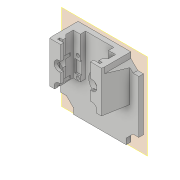
# Autodesk Inventor part: 50_Cube_Insert_Thorlabs
Saved by Autodesk Inventor 2019 (Build 230136000, 136)
## iProperties
Created: 2019-07-01
Part Number: 50_Cube_Insert_Thorlabs
Material: Generic
Document SubType Name: Modeling
Designer: diederichbenedict
Density: 1 g/cm^3
Appearance: Default
Author: diederichbenedict
Autodesk Inventor part; units mm, degrees
ref_plane "YZ Plane" through (0, 0, 0) normal (1, 0, 0) x (0, 1, 0)
ref_plane "XZ Plane" through (0, 0, 0) normal (0, 1, 0) x (-1, 0, 0)
ref_plane "Work Plane1" through (0, 0, 10) normal (0, 0, 1) x (1, 0, 0)
sketch "Sketch1" plane through (0, 0, 10) normal (0, 0, 1) x (1, 0, 0)
  line L0 (-4.0299, -0.3538) -> (-2.2322, 1.4439) construction
  arc A0 (-1.4439, 2.2322) -> (-2.2322, 1.4439) centre (-0.9299, 0.9299) ccw construction
  line L1 (-1.4439, 2.2322) -> (0.3538, 4.0299) construction
  line L2 (-37.8299, 42.2137) -> (-37.8299, 45.8299) construction
  line L3 (-37.8299, 45.8299) -> (-4.0299, 45.8299) construction
  line L4 (-4.0299, 45.8299) -> (-4.0299, 42.2137) construction
  line L5 (-4.0299, 4.0299) -> (0.3538, 4.0299) projected
  circle A1 centre (-20.9299, 20.9299) radius 17.5 projected
  line L6 (-20.9299, 58.9723) -> (17.1124, 20.9299) construction
  line L7 (17.1124, 20.9299) -> (-20.9299, -17.1124) construction
  line L8 (-20.9299, -17.1124) -> (-58.9723, 20.9299) construction
  line L9 (-58.9723, 20.9299) -> (-20.9299, 58.9723) construction
  line L10 (-20.9299, 58.9723) -> (-20.9299, -17.1124) construction
  line L11 (17.1124, 20.9299) -> (-58.9723, 20.9299) construction
  line L12 (-20.9299, 58.9723) -> (32.8701, 58.9723) construction
  line L13 (-43.4299, 43.4299) -> (1.5701, 43.4299) construction
  line L14 (1.5701, 43.4299) -> (1.5701, -1.5701) construction
  line L15 (1.5701, -1.5701) -> (-43.4299, -1.5701) construction
  line L16 (-43.4299, -1.5701) -> (-43.4299, 43.4299) construction
  line L17 (-43.4299, 43.4299) -> (1.5701, -1.5701) construction
  line L18 (1.5701, 43.4299) -> (-43.4299, -1.5701) construction
  line L19 (-43.4299, 5.3876) -> (-43.4299, 36.4723)
  line L20 (-43.4299, 36.4723) -> (-36.4723, 43.4299)
  line L21 (-36.4723, 43.4299) -> (-5.3876, 43.4299)
  line L22 (-5.3876, 43.4299) -> (1.5701, 36.4723)
  line L23 (1.5701, 36.4723) -> (1.5701, 5.3876)
  line L24 (1.5701, 5.3876) -> (-5.3876, -1.5701)
  line L25 (-5.3876, -1.5701) -> (-36.4723, -1.5701)
  line L26 (-36.4723, -1.5701) -> (-43.4299, 5.3876)
  line L27 (-4.0299, 42.2137) -> (-37.8299, 42.2137) projected
  line L28 (-4.0299, -0.3538) -> (-4.0299, 4.0299) projected
  circle A2 centre (-20.9299, 20.9299) radius 7.0417
  point P0 (-37.8299, 4.0299)
  dimension "d18" = 53.8
  dimension "d19" = 45
  dimension "d20" = 53.8
  dimension "d21" = 45
  dimension "d22" = 45
  constraints: 42 end point, 15 point on line, 5 midpoint, 4 parallel, 3 perpendicular, 2 horizontal, 1 centre point, 1 coincident, 1 equal length
  measures "d18" distance of L6.start L6.end
  measures "d19" angle of L6 L12
  measures "d20" distance of L6.end L7.end
  measures "d21" distance of L14.end L15.end
  measures "d22" distance of L13.end L14.end
extrude "Extrusion1" add sketch "Sketch1" along normal blind 3 contours L28 L24 L25 L26 L19 L20 L27 L22 L23 L5 | L5 L24 L28 | L27 L20 L21 L22 | A1
sketch "Sketch3" plane through (0, 0, 10) normal (0, 0, -1) x (-1, 0, 0)
  line L0 (37.8299, -0.4701) -> (37.8299, 4.0299) construction
  line L1 (4.0299, 4.0299) -> (4.0299, -0.4701) construction
  line L2 (37.8299, -0.4701) -> (37.8299, 1.1886) construction
  line L3 (4.0299, -3.9701) -> (4.0299, -0.3538) construction
  line L4 (45.8299, 4.0299) -> (42.2137, 4.0299) construction
  line L5 (-0.3538, 4.0299) -> (-3.9701, 4.0299) construction
  line L6 (-3.9701, 37.8299) -> (-0.3538, 37.8299) construction
  line L7 (4.0299, 42.2137) -> (4.0299, 45.8299) construction
  line L8 (37.8299, 45.8299) -> (37.8299, 42.2137) construction
  line L9 (42.2137, 37.8299) -> (45.8299, 37.8299) construction
  line L10 (37.8299, 37.7299) -> (45.8299, 37.7299)
  line L11 (45.8299, 37.7299) -> (45.8299, 4.1299)
  line L12 (45.8299, 4.1299) -> (37.8299, 4.1299)
  line L13 (37.8299, 4.1299) -> (37.8299, 37.7299)
  line L14 (37.7299, 4.0299) -> (4.1299, 4.0299)
  line L15 (4.1299, 4.0299) -> (4.1299, -3.9701)
  line L16 (4.1299, -3.9701) -> (37.7299, -3.9701)
  line L17 (37.7299, -3.9701) -> (37.7299, 4.0299)
  line L18 (4.0299, 4.1299) -> (-3.9701, 4.1299)
  line L19 (-3.9701, 4.1299) -> (-3.9701, 37.7299)
  line L20 (-3.9701, 37.7299) -> (4.0299, 37.7299)
  line L21 (4.0299, 37.7299) -> (4.0299, 4.1299)
  line L22 (4.1299, 37.8299) -> (37.7299, 37.8299)
  line L23 (37.7299, 37.8299) -> (37.7299, 45.8299)
  line L24 (37.7299, 45.8299) -> (4.1299, 45.8299)
  line L25 (4.1299, 45.8299) -> (4.1299, 37.8299)
  point P0 (0, 0)
  dimension "d23" = 0.1
  dimension "d24" = 0.1
  dimension "d25" = 0.1
  dimension "d26" = 0.1
  dimension "d27" = 0.1
  constraints: 32 end point, 8 parallel, 4 horizontal, 4 perpendicular, 3 point on line
  measures "d23" distance between parallel lines of L8 L23
  measures "d24" distance between parallel lines of L7 L25
  measures "d25" distance between parallel lines of L6 L20
  measures "d26" distance between parallel lines of L5 L18
  measures "d27" distance between parallel lines of L1 L15
extrude "Extrusion3" add sketch "Sketch3" against normal up to surface (3 mm away)
sketch "Sketch4" plane through (0, 0, 13) normal (0, 0, 1) x (1, 0, 0)
  line L0 (-33.4299, 35.4299) -> (-33.4299, 11.4299) construction
  line L1 (-33.4299, 11.4299) -> (-8.4299, 11.4299) construction
  line L2 (-8.4299, 11.4299) -> (-8.4299, 35.4299) construction
  line L3 (-8.4299, 35.4299) -> (-33.4299, 35.4299) construction
  circle A0 centre (-10.4299, 33.4299) radius 1.05 construction
  circle A1 centre (-10.4299, 20.9299) radius 1.05 construction
  circle A2 centre (-31.4299, 20.9299) radius 1.05 construction
  circle A3 centre (-31.4299, 33.4299) radius 1.05 construction
  line L4 (-15.4299, 29.8299) -> (-12.4299, 29.8299) construction
  line L5 (-15.4299, 31.8299) -> (-15.4299, 29.8299) construction
  line L6 (-12.4299, 31.8299) -> (-15.4299, 31.8299) construction
  line L7 (-12.4299, 29.8299) -> (-12.4299, 31.8299) construction
  line L8 (-8.4299, 35.4299) -> (-11.9299, 35.4299)
  line L9 (-11.9299, 35.4299) -> (-11.9299, 19.4299)
  line L10 (-11.9299, 19.4299) -> (-8.4299, 19.4299)
  line L11 (-8.4299, 19.4299) -> (-8.4299, 35.4299)
  line L12 (-33.4299, 35.4299) -> (-29.9299, 35.4299)
  line L13 (-29.9299, 35.4299) -> (-29.9299, 19.4299)
  line L14 (-29.9299, 19.4299) -> (-33.4299, 19.4299)
  line L15 (-33.4299, 19.4299) -> (-33.4299, 35.4299)
  line L16 (-33.4299, 35.4299) -> (-37.4299, 35.4299)
  line L17 (-37.4299, 35.4299) -> (-37.4299, 19.4299)
  line L18 (-37.4299, 19.4299) -> (-33.4299, 19.4299)
  line L19 (-33.4299, 19.4299) -> (-33.4299, 35.4299)
  line L20 (-8.4299, 35.4299) -> (-4.4299, 35.4299)
  line L21 (-4.4299, 35.4299) -> (-4.4299, 19.4299)
  line L22 (-4.4299, 19.4299) -> (-8.4299, 19.4299)
  line L23 (-8.4299, 19.4299) -> (-8.4299, 35.4299)
  point P0 (0, 0)
  dimension "d30" = 3.5
  dimension "d31" = 16
  dimension "d32" = 3.5
  dimension "d37" = 4
  dimension "d38" = 4
  constraints: 32 end point, 8 parallel, 4 horizontal, 4 perpendicular, 2 point on line
  measures "d30" distance of L10.end L9.end
  measures "d31" distance of L9.end L8.end
  measures "d32" distance of L13.end L14.end
  measures "d37" distance of L18.end L17.end
  measures "d38" distance of L21.end L22.end
ref_plane "Work Plane3" through (-33.4299, 11.4299, 16.4) normal (0, 0, -1) x (0, 1, 0)
extrude "Extrusion4" add sketch "Sketch4" along normal up to surface (3.4 mm away)
sketch "Sketch5" plane through (-11.9299, 35.4299, 16.4) normal (0, 0, 1) x (1, 0, 0)
  circle A0 centre (1.5, -14.5) radius 1.05 projected
  circle A1 centre (1.5, -2) radius 1.05 projected
  circle A2 centre (-19.5, -2) radius 1.05 projected
  circle A3 centre (-19.5, -14.5) radius 1.05 projected
  point P0 (11.9299, -35.4299)
extrude "Extrusion5" cut sketch "Sketch5" against normal through all
sketch "Sketch7" plane through (-37.4299, 35.4299, 13) normal (0, 1, 0) x (1, 0, 0)
  line L0 (4.95, -3.4) -> (4.95, 3) projected
  line L1 (7.5, -3.4) -> (0, -3.4) projected
  line L2 (7.5, 0) -> (7.5, -3.4) projected
  line L3 (0, 0) -> (7.5, 0) projected
  line L4 (0, 0) -> (0, -3.4) projected
  line L5 (33, -3.4) -> (25.5, -3.4) projected
  line L6 (33, 0) -> (33, -3.4) projected
  line L7 (25.5, 0) -> (33, 0) projected
  line L8 (25.5, 0) -> (25.5, -3.4) projected
  line L9 (0, -3.4) -> (7.5, -3.4) projected
  line L10 (0, -3.4) -> (3, -3.4)
  line L11 (3, -3.4) -> (3, -13.4)
  line L12 (3, -13.4) -> (0, -13.4)
  line L13 (0, -13.4) -> (0, -3.4)
  line L14 (33, -3.4) -> (30, -3.4)
  line L15 (30, -3.4) -> (30, -13.4)
  line L16 (30, -13.4) -> (33, -13.4)
  line L17 (33, -13.4) -> (33, -3.4)
  line L18 (0, -13.4) -> (7, -13.4)
  line L19 (7, -13.4) -> (7, -15.4)
  line L20 (7, -15.4) -> (0, -15.4)
  line L21 (0, -15.4) -> (0, -13.4)
  line L22 (33, -13.4) -> (26, -13.4)
  line L23 (26, -13.4) -> (26, -15.4)
  line L24 (26, -15.4) -> (33, -15.4)
  line L25 (33, -15.4) -> (33, -13.4)
  line L26 (3, -12) -> (5, -12)
  line L27 (5, -12) -> (5, -10)
  line L28 (5, -10) -> (3, -10)
  line L29 (3, -10) -> (3, -12)
  line L30 (30, -12) -> (28, -12)
  line L31 (28, -12) -> (28, -10)
  line L32 (28, -10) -> (30, -10)
  line L33 (30, -10) -> (30, -12)
  line L34 (5, -10) -> (3, -8)
  line L35 (5, -10) -> (7.8284, -10) construction
  line L36 (28, -10) -> (30, -8)
  line L37 (0, -15.4) -> (-2.7154, 0)
  line L38 (-4.7423, 0) -> (-0.3, 0) projected
  line L39 (0, -15.4) -> (15.6376, -15.4) construction
  line L40 (-2.7154, 0) -> (0, 0)
  line L41 (0, -15.4) -> (0, 0)
  line L42 (33, -15.4) -> (35.7154, 0)
  line L43 (33, -15.4) -> (48.6376, -15.4) construction
  line L44 (35.7154, 0) -> (33, 0)
  line L45 (37.7423, 0) -> (33.3, 0) projected
  line L46 (33, -15.4) -> (33, 0)
  point P0 (37.4299, 13)
  dimension "d39" = 3
  dimension "d40" = 10
  dimension "d41" = 3
  dimension "d42" = 7
  dimension "d43" = 2
  dimension "d44" = 7
  dimension "d47" = 27
  dimension "d48" = 1.4
  dimension "d49" = 2
  dimension "d50" = 2
  dimension "d51" = 2
  dimension "d52" = 135
  dimension "d53" = 100
  dimension "d54" = 80
  constraints: 70 end point, 12 parallel, 10 point on line, 9 horizontal, 8 perpendicular, 3 equal length, 2 collinear
  measures "d39" distance of L11.end L12.end
  measures "d40" distance of L10.end L11.end
  measures "d41" distance of L16.end L15.end
  measures "d42" distance of L19.end L20.end
  measures "d43" distance of L18.end L19.end
  measures "d44" distance of L24.end L23.end
  measures "d47" distance between parallel lines of L15 L11
  measures "d48" distance between parallel lines of L18 L26
  measures "d49" distance between parallel lines of L27 L11
  measures "d50" distance between parallel lines of L33 L31
  measures "d51" distance between parallel lines of L26 L28
  measures "d52" angle of L35 L34
  measures "d53" angle of L39 L37
  measures "d54" angle of L43 L42
extrude "Extrusion6" add sketch "Sketch7" against normal up to surface (16 mm away) contours L11 L12 L13 L1 | L4 L13 L21 L37 L38 L40 | L34 L28 L11 | L12 L18 L19 L20 L21 | L28 L27 L26 L11 | L17 L16 L15 L5 | L6 L44 L42 L25 L17 | L25 L24 L23 L22 L16 | L15 L32 L36 | L15 L30 L31 L32
sketch "Sketch8" plane through (-29.9299, 35.4299, 16.4) normal (0, 1, 0) x (1, 0, 0)
  line L0 (0, 0) -> (-4.5, 0) projected
  line L1 (0, 3.4) -> (0, 0) projected
  line L2 (-10.2154, 3.4) -> (0, 3.4) projected
  line L3 (-10.2154, 3.4) -> (-7.5, -12) projected
  line L4 (-7.5, -12) -> (-0.5, -12) projected
  line L5 (-0.5, -12) -> (-0.5, -10) projected
  line L6 (-0.5, -10) -> (-4.5, -10) projected
  line L7 (-4.5, -10) -> (-4.5, -8.6) projected
  line L8 (-4.5, -8.6) -> (-2.5, -8.6) projected
  line L9 (-2.5, -8.6) -> (-2.5, -6.6) projected
  line L10 (-2.5, -6.6) -> (-4.5, -4.6) projected
  line L11 (-4.5, -4.6) -> (-4.5, 0) projected
  line L12 (18, 3.4) -> (28.2154, 3.4) projected
  line L13 (18, 3.4) -> (18, 0) projected
  line L14 (22.5, 0) -> (18, 0) projected
  line L15 (22.5, 0) -> (22.5, -4.6) projected
  line L16 (22.5, -4.6) -> (20.5, -6.6) projected
  line L17 (20.5, -6.6) -> (20.5, -8.6) projected
  line L18 (20.5, -8.6) -> (22.5, -8.6) projected
  line L19 (22.5, -8.6) -> (22.5, -10) projected
  line L20 (22.5, -10) -> (18.5, -10) projected
  line L21 (18.5, -10) -> (18.5, -12) projected
  line L22 (18.5, -12) -> (25.5, -12) projected
  line L23 (25.5, -12) -> (28.2154, 3.4) projected
  point P0 (29.9299, 16.4)
extrude "Extrusion7" add sketch "Sketch8" along normal up to surface (10.4 mm away)
sketch "Sketch9" plane through (-37.7299, 45.8299, 13) normal (0, 0, -1) x (-1, 0, 0)
  line L0 (0, -3.6577) -> (2.4154, -6.0731) projected
  line L1 (2.4154, -6.0731) -> (2.4154, 0) projected
  line L2 (2.4154, 0) -> (0, 0) projected
  line L3 (0, -3.6577) -> (0, 0) projected
  line L4 (-33.6, 0) -> (-33.6, -3.6577) projected
  line L5 (-33.6, 0) -> (-36.0154, 0) projected
  line L6 (-36.0154, -6.0731) -> (-36.0154, 0) projected
  line L7 (-36.0154, -6.0731) -> (-33.6, -3.6577) projected
  point P0 (-37.7299, -45.8299)
extrude "Extrusion8" cut sketch "Sketch9" against normal through all
sketch "Sketch10" plane through (-29.9299, 19.4299, 16.4) normal (0, 0, 1) x (1, 0, 0)
  line L0 (0, 26.4) -> (0, 0) projected
  line L1 (18, 0) -> (18, 26.4) projected
  line L2 (-3.3664, 3.2942) -> (21.6336, 3.2942)
  line L3 (21.6336, 3.2942) -> (21.6336, 11.2942)
  line L4 (21.6336, 11.2942) -> (-3.3664, 11.2942)
  line L5 (-3.3664, 11.2942) -> (-3.3664, 3.2942)
  line L6 (-3.3664, 3.2942) -> (21.6336, 11.2942) construction
  line L7 (21.6336, 3.2942) -> (-3.3664, 11.2942) construction
  point P0 (29.9299, -19.4299)
  point P1 (9.1336, 7.2942)
  dimension "d59" = 25
  dimension "d60" = 8
  constraints: 12 end point, 2 midpoint, 2 parallel, 1 horizontal, 1 perpendicular
  measures "d59" distance of L4.end L3.end
  measures "d60" distance of L3.end L2.end
extrude "Extrusion9" cut sketch "Sketch10" against normal blind 1
sketch "Sketch11" plane through (-37.4299, 19.4299, 28.4) normal (0, 0, 1) x (1, 0, 0)
  line L0 (0, 0) -> (7, 0) projected
  line L1 (7, 0) -> (7, 26.4) projected
  line L2 (7, 26.4) -> (0, 26.4) projected
  line L3 (0, 26.4) -> (0, 0) projected
  line L4 (26, 0) -> (33, 0) projected
  line L5 (33, 0) -> (33, 26.4) projected
  line L6 (33, 26.4) -> (26, 26.4) projected
  line L7 (26, 0) -> (26, 26.4) projected
  circle A0 centre (16.5, 1.5) radius 7.0417 projected
  circle A1 centre (6, 1.5) radius 1.05 construction
  circle A2 centre (6, 14) radius 1.05 construction
  line L8 (27, 1.5) -> (6, 1.5) construction
  line L9 (27, 4.6642) -> (6, 4.6642)
  line L10 (6, -1.6642) -> (27, -1.6642)
  arc A3 (27, -1.6642) -> (27, 4.6642) centre (27, 1.5) ccw
  arc A4 (6, 4.6642) -> (6, -1.6642) centre (6, 1.5) ccw
  line L11 (27, 14) -> (6, 14) construction
  line L12 (27, 17.1642) -> (6, 17.1642)
  line L13 (6, 10.8358) -> (27, 10.8358)
  arc A5 (27, 10.8358) -> (27, 17.1642) centre (27, 14) ccw
  arc A6 (6, 17.1642) -> (6, 10.8358) centre (6, 14) ccw
  point P0 (37.4299, -19.4299)
  point P1 (16.5, 14)
  constraints: 16 end point, 8 point on circle, 8 tangent, 4 centre point, 3 parallel, 2 midpoint, 1 horizontal
extrude "Extrusion10" cut sketch "Sketch11" against normal blind 10 contours A4 L9 L1 L0 | L0 L1 L9 A0 L10 A4 | A0 L9 L10 | L12 L7 L13 L1 | L1 L13 A6 L12 | A0 L9 L7 L4 A3 L10 | L12 A5 L13 L7 | L9 A3 L4 L7
body "Solid1"
